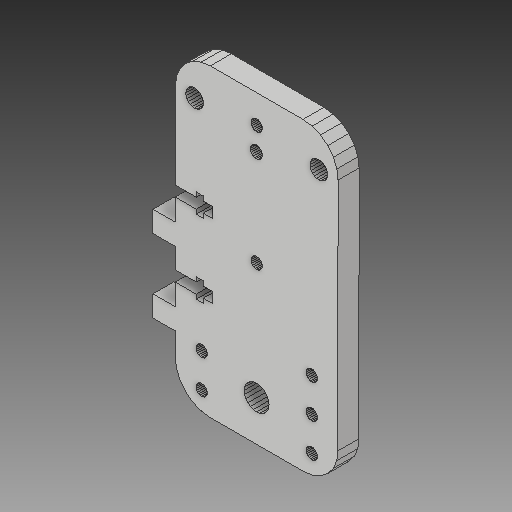
# Autodesk Inventor part: Hotend Rear Plate
Saved by Autodesk Inventor 2018 (Build 220112000, 112)
## iProperties
Created: 2016-07-21
Part Number: Hotend Rear Plate
Material: Generic
Document SubType Name: Modeling
Designer: User
Density: 1 g/cm^3
Appearance: Default
Mass: 22.8584 g
Surface Area: 103.9 cm^2
Volume: 22.8584 cm^3
Author: User
Autodesk Inventor part; units mm, degrees
ref_plane "YZ Plane" through (0, 0, 0) normal (1, 0, 0) x (0, 1, 0)
ref_plane "XZ Plane" through (0, 0, 0) normal (0, 1, 0) x (-1, 0, 0)
ref_plane "XY Plane" through (0, 0, 0) normal (0, 0, 1) x (1, 0, 0)
sketch "Sketch1" plane through (0, 0, 0) normal (0, 0, 1) x (1, 0, 0)
  line L0 (182.3386, 395.2631) -> (182.1886, 395.6381)
  line L1 (182.1886, 395.6381) -> (181.9387, 395.9882)
  line L2 (181.9387, 395.9882) -> (181.6139, 396.2384)
  line L3 (181.6139, 396.2384) -> (181.2138, 396.3883)
  line L4 (181.2138, 396.3883) -> (180.8138, 396.4383)
  line L5 (180.8138, 396.4383) -> (180.3888, 396.3883)
  line L6 (180.3888, 396.3883) -> (180.0139, 396.2382)
  line L7 (180.0139, 396.2382) -> (179.6637, 395.9884)
  line L8 (179.6637, 395.9884) -> (179.4135, 395.6385)
  line L9 (179.4135, 395.6385) -> (179.2636, 395.2635)
  line L10 (179.2636, 395.2635) -> (179.2135, 394.8385)
  line L11 (179.2135, 394.8385) -> (179.2636, 394.4385)
  line L12 (179.2636, 394.4385) -> (179.4135, 394.0385)
  line L13 (179.4135, 394.0385) -> (179.6635, 393.7135)
  line L14 (179.6635, 393.7135) -> (180.0134, 393.4633)
  line L15 (180.0134, 393.4633) -> (180.3884, 393.3133)
  line L16 (180.3884, 393.3133) -> (180.8134, 393.2387)
  line L17 (180.8134, 393.2387) -> (181.2132, 393.3133)
  line L18 (181.2132, 393.3133) -> (181.6132, 393.4633)
  line L19 (181.6132, 393.4633) -> (181.9382, 393.7132)
  line L20 (181.9382, 393.7132) -> (182.1884, 394.0381)
  line L21 (182.1884, 394.0381) -> (182.3384, 394.4382)
  line L22 (182.3384, 394.4382) -> (182.4134, 394.8381)
  line L23 (182.4134, 394.8381) -> (182.3386, 395.2631)
  line L24 (182.3403, 404.8886) -> (182.1904, 405.2886)
  line L25 (182.1904, 405.2886) -> (181.9404, 405.6136)
  line L26 (181.9404, 405.6136) -> (181.6156, 405.8637)
  line L27 (181.6156, 405.8637) -> (181.2156, 406.039)
  line L28 (181.2156, 406.039) -> (180.8157, 406.0889)
  line L29 (180.8157, 406.0889) -> (180.3907, 406.0389)
  line L30 (180.3907, 406.0389) -> (180.0156, 405.864)
  line L31 (180.0156, 405.864) -> (179.6654, 405.6142)
  line L32 (179.6654, 405.6142) -> (179.4153, 405.2893)
  line L33 (179.4153, 405.2893) -> (179.2653, 404.8893)
  line L34 (179.2653, 404.8893) -> (179.2154, 404.4893)
  line L35 (179.2154, 404.4893) -> (179.2654, 404.0643)
  line L36 (179.2654, 404.0643) -> (179.4155, 403.6893)
  line L37 (179.4155, 403.6893) -> (179.6654, 403.3643)
  line L38 (179.6654, 403.3643) -> (180.0155, 403.0893)
  line L39 (180.0155, 403.0893) -> (180.3905, 402.9393)
  line L40 (180.3905, 402.9393) -> (180.8155, 402.8893)
  line L41 (180.8155, 402.8893) -> (181.2154, 402.9393)
  line L42 (181.2154, 402.9393) -> (181.6155, 403.0893)
  line L43 (181.6155, 403.0893) -> (181.9402, 403.3637)
  line L44 (181.9402, 403.3637) -> (182.1903, 403.6886)
  line L45 (182.1903, 403.6886) -> (182.3403, 404.0636)
  line L46 (182.3403, 404.0636) -> (182.4149, 404.489)
  line L47 (182.4149, 404.489) -> (182.3403, 404.8886)
  line L48 (199.9396, 401.6874) -> (199.5895, 402.5623)
  line L49 (199.5895, 402.5623) -> (199.0399, 403.2877)
  line L50 (199.0399, 403.2877) -> (198.2902, 403.8631)
  line L51 (198.2902, 403.8631) -> (197.4404, 404.2135)
  line L52 (197.4404, 404.2135) -> (196.5154, 404.3389)
  line L53 (196.5154, 404.3389) -> (195.5904, 404.2139)
  line L54 (195.5904, 404.2139) -> (194.7402, 403.8645)
  line L55 (194.7402, 403.8645) -> (194.0152, 403.2894)
  line L56 (194.0152, 403.2894) -> (193.4403, 402.5643)
  line L57 (193.4403, 402.5643) -> (193.0904, 401.6893)
  line L58 (193.0904, 401.6893) -> (192.9654, 400.7893)
  line L59 (192.9654, 400.7893) -> (193.0904, 399.8643)
  line L60 (193.0904, 399.8643) -> (193.4398, 399.0141)
  line L61 (193.4398, 399.0141) -> (194.0143, 398.2637)
  line L62 (194.0143, 398.2637) -> (194.739, 397.7132)
  line L63 (194.739, 397.7132) -> (195.5888, 397.3628)
  line L64 (195.5888, 397.3628) -> (196.5137, 397.2373)
  line L65 (196.5137, 397.2373) -> (197.4387, 397.3624)
  line L66 (197.4387, 397.3624) -> (198.289, 397.7118)
  line L67 (198.289, 397.7118) -> (199.0391, 398.2616)
  line L68 (199.0391, 398.2616) -> (199.5895, 399.0113)
  line L69 (199.5895, 399.0113) -> (199.9399, 399.8611)
  line L70 (199.9399, 399.8611) -> (200.0655, 400.7867)
  line L71 (200.0655, 400.7867) -> (199.9396, 401.6874)
  line L72 (213.7901, 404.8893) -> (213.6401, 405.2893)
  line L73 (213.6401, 405.2893) -> (213.3654, 405.6144)
  line L74 (213.3654, 405.6144) -> (213.0405, 405.8645)
  line L75 (213.0405, 405.8645) -> (212.6655, 406.0395)
  line L76 (212.6655, 406.0395) -> (212.2405, 406.0895)
  line L77 (212.2405, 406.0895) -> (211.8406, 406.0395)
  line L78 (211.8406, 406.0395) -> (211.4407, 405.8641)
  line L79 (211.4407, 405.8641) -> (211.1157, 405.6141)
  line L80 (211.1157, 405.6141) -> (210.8656, 405.2892)
  line L81 (210.8656, 405.2892) -> (210.6903, 404.8893)
  line L82 (210.6903, 404.8893) -> (210.6404, 404.4893)
  line L83 (210.6404, 404.4893) -> (210.6904, 404.0643)
  line L84 (210.6904, 404.0643) -> (210.8653, 403.6893)
  line L85 (210.8653, 403.6893) -> (211.1153, 403.3642)
  line L86 (211.1153, 403.3642) -> (211.4397, 403.0889)
  line L87 (211.4397, 403.0889) -> (211.8398, 402.9389)
  line L88 (211.8398, 402.9389) -> (212.2397, 402.889)
  line L89 (212.2397, 402.889) -> (212.6648, 402.939)
  line L90 (212.6648, 402.939) -> (213.0397, 403.089)
  line L91 (213.0397, 403.089) -> (213.3649, 403.3639)
  line L92 (213.3649, 403.3639) -> (213.6402, 403.6895)
  line L93 (213.6402, 403.6895) -> (213.7901, 404.0645)
  line L94 (213.7901, 404.0645) -> (213.8401, 404.4892)
  line L95 (213.8401, 404.4892) -> (213.7901, 404.8893)
  line L96 (213.7902, 395.264) -> (213.6401, 395.639)
  line L97 (213.6401, 395.639) -> (213.3655, 395.989)
  line L98 (213.3655, 395.989) -> (213.0406, 396.2391)
  line L99 (213.0406, 396.2391) -> (212.6656, 396.3891)
  line L100 (212.6656, 396.3891) -> (212.2406, 396.4391)
  line L101 (212.2406, 396.4391) -> (211.8407, 396.3891)
  line L102 (211.8407, 396.3891) -> (211.4406, 396.2391)
  line L103 (211.4406, 396.2391) -> (211.1156, 395.9892)
  line L104 (211.1156, 395.9892) -> (210.8654, 395.6393)
  line L105 (210.8654, 395.6393) -> (210.6904, 395.2643)
  line L106 (210.6904, 395.2643) -> (210.6404, 394.8393)
  line L107 (210.6404, 394.8393) -> (210.6904, 394.4393)
  line L108 (210.6904, 394.4393) -> (210.8658, 394.0395)
  line L109 (210.8658, 394.0395) -> (211.1158, 393.7145)
  line L110 (211.1158, 393.7145) -> (211.4407, 393.4643)
  line L111 (211.4407, 393.4643) -> (211.8407, 393.3144)
  line L112 (211.8407, 393.3144) -> (212.2407, 393.2393)
  line L113 (212.2407, 393.2393) -> (212.6656, 393.3141)
  line L114 (212.6656, 393.3141) -> (213.0406, 393.4641)
  line L115 (213.0406, 393.4641) -> (213.3656, 393.7141)
  line L116 (213.3656, 393.7141) -> (213.6403, 394.039)
  line L117 (213.6403, 394.039) -> (213.7903, 394.439)
  line L118 (213.7903, 394.439) -> (213.8402, 394.839)
  line L119 (213.8402, 394.839) -> (213.7902, 395.264)
  line L120 (213.7903, 414.5391) -> (213.6402, 414.9141)
  line L121 (213.6402, 414.9141) -> (213.3656, 415.2641)
  line L122 (213.3656, 415.2641) -> (213.0407, 415.5143)
  line L123 (213.0407, 415.5143) -> (212.6657, 415.6642)
  line L124 (212.6657, 415.6642) -> (212.2407, 415.7143)
  line L125 (212.2407, 415.7143) -> (211.8408, 415.6642)
  line L126 (211.8408, 415.6642) -> (211.4407, 415.5143)
  line L127 (211.4407, 415.5143) -> (211.1157, 415.2643)
  line L128 (211.1157, 415.2643) -> (210.8654, 414.9143)
  line L129 (210.8654, 414.9143) -> (210.6904, 414.5393)
  line L130 (210.6904, 414.5393) -> (210.6404, 414.1143)
  line L131 (210.6404, 414.1143) -> (210.6904, 413.7143)
  line L132 (210.6904, 413.7143) -> (210.8658, 413.3145)
  line L133 (210.8658, 413.3145) -> (211.1158, 412.9894)
  line L134 (211.1158, 412.9894) -> (211.4407, 412.7393)
  line L135 (211.4407, 412.7393) -> (211.8406, 412.5641)
  line L136 (211.8406, 412.5641) -> (212.2406, 412.5141)
  line L137 (212.2406, 412.5141) -> (212.6656, 412.5641)
  line L138 (212.6656, 412.5641) -> (213.0407, 412.7391)
  line L139 (213.0407, 412.7391) -> (213.3657, 412.989)
  line L140 (213.3657, 412.989) -> (213.6404, 413.314)
  line L141 (213.6404, 413.314) -> (213.7904, 413.7139)
  line L142 (213.7904, 413.7139) -> (213.8403, 414.114)
  line L143 (213.8403, 414.114) -> (213.7903, 414.5391)
  line L144 (198.0658, 434.4891) -> (197.8903, 434.889)
  line L145 (197.8903, 434.889) -> (197.6403, 435.214)
  line L146 (197.6403, 435.214) -> (197.3154, 435.4641)
  line L147 (197.3154, 435.4641) -> (196.9404, 435.6141)
  line L148 (196.9404, 435.6141) -> (196.5154, 435.6641)
  line L149 (196.5154, 435.6641) -> (196.1154, 435.6141)
  line L150 (196.1154, 435.6141) -> (195.7154, 435.4641)
  line L151 (195.7154, 435.4641) -> (195.3904, 435.2141)
  line L152 (195.3904, 435.2141) -> (195.1403, 434.8893)
  line L153 (195.1403, 434.8893) -> (194.9903, 434.4893)
  line L154 (194.9903, 434.4893) -> (194.9404, 434.0893)
  line L155 (194.9404, 434.0893) -> (194.9904, 433.6643)
  line L156 (194.9904, 433.6643) -> (195.1405, 433.2893)
  line L157 (195.1405, 433.2893) -> (195.3905, 432.9643)
  line L158 (195.3905, 432.9643) -> (195.7153, 432.7142)
  line L159 (195.7153, 432.7142) -> (196.1152, 432.5389)
  line L160 (196.1152, 432.5389) -> (196.5152, 432.489)
  line L161 (196.5152, 432.489) -> (196.9402, 432.539)
  line L162 (196.9402, 432.539) -> (197.3153, 432.7139)
  line L163 (197.3153, 432.7139) -> (197.6403, 432.9639)
  line L164 (197.6403, 432.9639) -> (197.8904, 433.2888)
  line L165 (197.8904, 433.2888) -> (198.0658, 433.6645)
  line L166 (198.0658, 433.6645) -> (198.1158, 434.0893)
  line L167 (198.1158, 434.0893) -> (198.0658, 434.4891)
  line L168 (198.0632, 461.9217) -> (197.8885, 462.3468)
  line L169 (197.8885, 462.3468) -> (197.6138, 462.697)
  line L170 (197.6138, 462.697) -> (197.2639, 462.9472)
  line L171 (197.2639, 462.9472) -> (196.864, 463.1224)
  line L172 (196.864, 463.1224) -> (196.4141, 463.1977)
  line L173 (196.4141, 463.1977) -> (195.9891, 463.123)
  line L174 (195.9891, 463.123) -> (195.5639, 462.9482)
  line L175 (195.5639, 462.9482) -> (195.2138, 462.6984)
  line L176 (195.2138, 462.6984) -> (194.9388, 462.3485)
  line L177 (194.9388, 462.3485) -> (194.7891, 461.9233)
  line L178 (194.7891, 461.9233) -> (194.7145, 461.4983)
  line L179 (194.7145, 461.4983) -> (194.7898, 461.0483)
  line L180 (194.7898, 461.0483) -> (194.9398, 460.6483)
  line L181 (194.9398, 460.6483) -> (195.2147, 460.2733)
  line L182 (195.2147, 460.2733) -> (195.5646, 460.0231)
  line L183 (195.5646, 460.0231) -> (195.9895, 459.8478)
  line L184 (195.9895, 459.8478) -> (196.4145, 459.7978)
  line L185 (196.4145, 459.7978) -> (196.8645, 459.8477)
  line L186 (196.8645, 459.8477) -> (197.2643, 460.0232)
  line L187 (197.2643, 460.0232) -> (197.6145, 460.273)
  line L188 (197.6145, 460.273) -> (197.8897, 460.6478)
  line L189 (197.8897, 460.6478) -> (198.0649, 461.0477)
  line L190 (198.0649, 461.0477) -> (198.1132, 461.4966)
  line L191 (198.1132, 461.4966) -> (198.0632, 461.9217)
  line L192 (198.0648, 468.489) -> (197.9148, 468.889)
  line L193 (197.9148, 468.889) -> (197.6401, 469.2141)
  line L194 (197.6401, 469.2141) -> (197.3152, 469.4642)
  line L195 (197.3152, 469.4642) -> (196.9402, 469.6142)
  line L196 (196.9402, 469.6142) -> (196.5158, 469.6887)
  line L197 (196.5158, 469.6887) -> (196.1158, 469.614)
  line L198 (196.1158, 469.614) -> (195.7157, 469.4641)
  line L199 (195.7157, 469.4641) -> (195.3907, 469.2141)
  line L200 (195.3907, 469.2141) -> (195.1406, 468.8892)
  line L201 (195.1406, 468.8892) -> (194.9653, 468.4893)
  line L202 (194.9653, 468.4893) -> (194.9154, 468.0893)
  line L203 (194.9154, 468.0893) -> (194.9654, 467.6643)
  line L204 (194.9654, 467.6643) -> (195.1403, 467.2893)
  line L205 (195.1403, 467.2893) -> (195.3901, 466.9391)
  line L206 (195.3901, 466.9391) -> (195.715, 466.689)
  line L207 (195.715, 466.689) -> (196.115, 466.539)
  line L208 (196.115, 466.539) -> (196.515, 466.4891)
  line L209 (196.515, 466.4891) -> (196.94, 466.5391)
  line L210 (196.94, 466.5391) -> (197.315, 466.6891)
  line L211 (197.315, 466.6891) -> (197.64, 466.9391)
  line L212 (197.64, 466.9391) -> (197.9148, 467.2888)
  line L213 (197.9148, 467.2888) -> (198.0648, 467.6639)
  line L214 (198.0648, 467.6639) -> (198.1148, 468.0889)
  line L215 (198.1148, 468.0889) -> (198.0648, 468.489)
  line L216 (216.6654, 466.6382) -> (216.4154, 467.2382)
  line L217 (216.4154, 467.2382) -> (216.0157, 467.7635)
  line L218 (216.0157, 467.7635) -> (215.4909, 468.1638)
  line L219 (215.4909, 468.1638) -> (214.8909, 468.4137)
  line L220 (214.8909, 468.4137) -> (214.2409, 468.4887)
  line L221 (214.2409, 468.4887) -> (213.5909, 468.4137)
  line L222 (213.5909, 468.4137) -> (212.9909, 468.1637)
  line L223 (212.9909, 468.1637) -> (212.4657, 467.7641)
  line L224 (212.4657, 467.7641) -> (212.0904, 467.2393)
  line L225 (212.0904, 467.2393) -> (211.8404, 466.6393)
  line L226 (211.8404, 466.6393) -> (211.7404, 465.9894)
  line L227 (211.7404, 465.9894) -> (211.8404, 465.3393)
  line L228 (211.8404, 465.3393) -> (212.0904, 464.7393)
  line L229 (212.0904, 464.7393) -> (212.4651, 464.2141)
  line L230 (212.4651, 464.2141) -> (212.9899, 463.8138)
  line L231 (212.9899, 463.8138) -> (213.5899, 463.5638)
  line L232 (213.5899, 463.5638) -> (214.2399, 463.4889)
  line L233 (214.2399, 463.4889) -> (214.8899, 463.5638)
  line L234 (214.8899, 463.5638) -> (215.4899, 463.8138)
  line L235 (215.4899, 463.8138) -> (216.0152, 464.2135)
  line L236 (216.0152, 464.2135) -> (216.4154, 464.7383)
  line L237 (216.4154, 464.7383) -> (216.6654, 465.3383)
  line L238 (216.6654, 465.3383) -> (216.7404, 465.9881)
  line L239 (216.7404, 465.9881) -> (216.6654, 466.6382)
  line L240 (181.2154, 466.6383) -> (180.9654, 467.2383)
  line L241 (180.9654, 467.2383) -> (180.5657, 467.7635)
  line L242 (180.5657, 467.7635) -> (180.041, 468.1638)
  line L243 (180.041, 468.1638) -> (179.441, 468.4137)
  line L244 (179.441, 468.4137) -> (178.7909, 468.4887)
  line L245 (178.7909, 468.4887) -> (178.1409, 468.4138)
  line L246 (178.1409, 468.4138) -> (177.5409, 468.1638)
  line L247 (177.5409, 468.1638) -> (177.0157, 467.7641)
  line L248 (177.0157, 467.7641) -> (176.6404, 467.2393)
  line L249 (176.6404, 467.2393) -> (176.3904, 466.6393)
  line L250 (176.3904, 466.6393) -> (176.2904, 465.9893)
  line L251 (176.2904, 465.9893) -> (176.3904, 465.3393)
  line L252 (176.3904, 465.3393) -> (176.6404, 464.7393)
  line L253 (176.6404, 464.7393) -> (177.0151, 464.2141)
  line L254 (177.0151, 464.2141) -> (177.5399, 463.8138)
  line L255 (177.5399, 463.8138) -> (178.1399, 463.5638)
  line L256 (178.1399, 463.5638) -> (178.7899, 463.4889)
  line L257 (178.7899, 463.4889) -> (179.4399, 463.5638)
  line L258 (179.4399, 463.5638) -> (180.0399, 463.8138)
  line L259 (180.0399, 463.8138) -> (180.5651, 464.2135)
  line L260 (180.5651, 464.2135) -> (180.9654, 464.7383)
  line L261 (180.9654, 464.7383) -> (181.2154, 465.3383)
  line L262 (181.2154, 465.3383) -> (181.2904, 465.9883)
  line L263 (181.2904, 465.9883) -> (181.2154, 466.6383)
  line L264 (219.4201, 468.7607) -> (218.4201, 471.1607)
  line L265 (218.4201, 471.1607) -> (216.82, 473.2356)
  line L266 (216.82, 473.2356) -> (214.7449, 474.8106)
  line L267 (214.7449, 474.8106) -> (212.3449, 475.8105)
  line L268 (212.3449, 475.8105) -> (209.7451, 476.1619)
  line L269 (209.7451, 476.1619) -> (183.2951, 476.1764)
  line L270 (183.2951, 476.1764) -> (180.7201, 475.8264)
  line L271 (180.7201, 475.8264) -> (178.2952, 474.8263)
  line L272 (178.2952, 474.8263) -> (176.2202, 473.2512)
  line L273 (176.2202, 473.2512) -> (174.6453, 471.1762)
  line L274 (174.6453, 471.1762) -> (173.6454, 468.7761)
  line L275 (173.6454, 468.7761) -> (173.2939, 466.1763)
  line L276 (173.2939, 466.1763) -> (173.2839, 447.8263)
  line L277 (173.2839, 447.8263) -> (173.2806, 441.7263)
  line L278 (173.2806, 441.7263) -> (179.2806, 441.723)
  line L279 (179.2806, 441.723) -> (179.2813, 442.9731)
  line L280 (179.2813, 442.9731) -> (181.2752, 442.972)
  line L281 (181.2752, 442.972) -> (181.2745, 441.7319)
  line L282 (181.2745, 441.7319) -> (183.9284, 441.7304)
  line L283 (183.9284, 441.7304) -> (183.9268, 438.7397)
  line L284 (183.9268, 438.7397) -> (181.2683, 438.7411)
  line L285 (181.2683, 438.7411) -> (181.2676, 437.4894)
  line L286 (181.2676, 437.4894) -> (179.2671, 437.4905)
  line L287 (179.2671, 437.4905) -> (179.2678, 438.7405)
  line L288 (179.2678, 438.7405) -> (173.2678, 438.7438)
  line L289 (173.2678, 438.7438) -> (173.2644, 432.5438)
  line L290 (173.2644, 432.5438) -> (166.9144, 432.5473)
  line L291 (166.9144, 432.5473) -> (166.9111, 426.5473)
  line L292 (166.9111, 426.5473) -> (173.2611, 426.5438)
  line L293 (173.2611, 426.5438) -> (173.2579, 420.7438)
  line L294 (173.2579, 420.7438) -> (179.258, 420.7405)
  line L295 (179.258, 420.7405) -> (179.2586, 421.9905)
  line L296 (179.2586, 421.9905) -> (181.2586, 421.9894)
  line L297 (181.2586, 421.9894) -> (181.2579, 420.7394)
  line L298 (181.2579, 420.7394) -> (183.8517, 420.738)
  line L299 (183.8517, 420.738) -> (183.8501, 417.7317)
  line L300 (183.8501, 417.7317) -> (181.2734, 417.7331)
  line L301 (181.2734, 417.7331) -> (181.2727, 416.4758)
  line L302 (181.2727, 416.4758) -> (179.2708, 416.4769)
  line L303 (179.2708, 416.4769) -> (179.2714, 417.7269)
  line L304 (179.2714, 417.7269) -> (173.2714, 417.7302)
  line L305 (173.2714, 417.7302) -> (173.2681, 411.6302)
  line L306 (173.2681, 411.6302) -> (166.9181, 411.6337)
  line L307 (166.9181, 411.6337) -> (166.9148, 405.6337)
  line L308 (166.9148, 405.6337) -> (173.2648, 405.6302)
  line L309 (173.2648, 405.6302) -> (173.2613, 399.2302)
  line L310 (173.2613, 399.2302) -> (173.6099, 396.63)
  line L311 (173.6099, 396.63) -> (174.6098, 394.23)
  line L312 (174.6098, 394.23) -> (176.1849, 392.155)
  line L313 (176.1849, 392.155) -> (178.2589, 390.5538)
  line L314 (178.2589, 390.5538) -> (180.6833, 389.5524)
  line L315 (180.6833, 389.5524) -> (183.2581, 389.2257)
  line L316 (183.2581, 389.2257) -> (192.9081, 389.2205)
  line L317 (192.9081, 389.2205) -> (200.0581, 389.2165)
  line L318 (200.0581, 389.2165) -> (209.7081, 389.2113)
  line L319 (209.7081, 389.2113) -> (212.3081, 389.5365)
  line L320 (212.3081, 389.5365) -> (214.7081, 390.5365)
  line L321 (214.7081, 390.5365) -> (216.783, 392.1366)
  line L322 (216.783, 392.1366) -> (218.3843, 394.2106)
  line L323 (218.3843, 394.2106) -> (219.3842, 396.6107)
  line L324 (219.3842, 396.6107) -> (219.7087, 399.2108)
  line L325 (219.7087, 399.2108) -> (219.7453, 466.1607)
  line L326 (219.7453, 466.1607) -> (219.4201, 468.7607)
  point P0 (0, 0)
  constraints: 654 end point, 134 parallel, 129 perpendicular, 1 collinear
extrude "Extrusion1" add sketch "Sketch1" along normal blind 6
body "Solid1"
